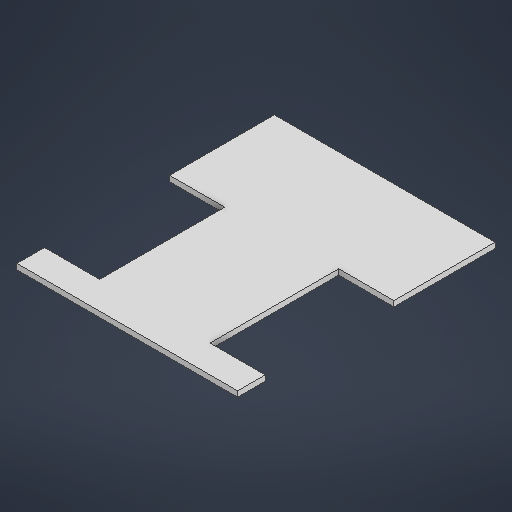
# Autodesk Inventor part: base
Saved by Autodesk Inventor 2026.1 (Build 301233000, 233)
## iProperties
Created: 2025-10-10
Part Number: base
Material: Generic
Document SubType Name: Modeling
Designer: plainakarin
Density: 1 g/cm^3
Appearance: Default
Author: plainakarin
Autodesk Inventor part; units mm, degrees
ref_plane "YZ Plane" through (0, 0, 0) normal (1, 0, 0) x (0, 1, 0)
ref_plane "XZ Plane" through (0, 0, 0) normal (0, 1, 0) x (-1, 0, 0)
ref_plane "XY Plane" through (0, 0, 0) normal (0, 0, 1) x (1, 0, 0)
sketch "Sketch2" plane through (0, 0, 0) normal (0, 1, 0) x (-1, 0, 0)
  line L0 (-60, 70) -> (60, 70)
  line L1 (60, -70) -> (-60, -70)
  line L2 (-60, 70) -> (60, -70) construction
  line L3 (60, 70) -> (-60, -70) construction
  line L4 (-60, 55) -> (-30, 55)
  line L5 (-30, 55) -> (-30, -15)
  line L6 (-30, -15) -> (-60, -15)
  line L7 (-60, -15) -> (-60, 55)
  line L8 (60, 55) -> (30, 55)
  line L9 (30, 55) -> (30, -13)
  line L10 (30, -13) -> (60, -13)
  line L11 (60, 70) -> (60, 55)
  line L12 (60, -13) -> (60, -70)
  line L13 (-60, -70) -> (-60, -15)
  line L14 (-60, 55) -> (-60, 70)
  point P0 (0, 0)
  dimension "d9" = 120
  dimension "d10" = 140
  dimension "d11" = 30
  dimension "d12" = 70
  dimension "d13" = 15
  dimension "d17" = 68
  dimension "d18" = 15
  constraints: 30 end point, 8 parallel, 4 perpendicular, 3 horizontal, 2 midpoint
  measures "d9" distance of L1.start L1.end
  measures "d10" distance of L0.end L1.start
  measures "d11" distance of L5.end L6.end
  measures "d12" distance of L4.end L5.end
  measures "d13" distance between parallel lines of L0 L4
  measures "d17" distance of L8.end L9.end
  measures "d18" distance between parallel lines of L8 L0
extrude "Extrusion2" add sketch "Sketch2" along normal blind 3 contours L0 L11 L8 L9 L10 L12 L1 L13 L6 L5 L4 L14
body "Solid2"
